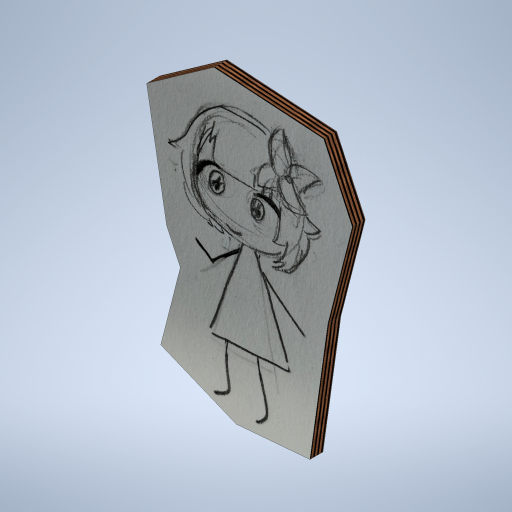
# Autodesk Inventor part: emu
Saved by Autodesk Inventor 2023 (Build 270158000, 158)
## iProperties
Created: 2024-07-02
Part Number: emu
Material: Generic
Document SubType Name: Modeling
Designer: Student-27
Density: 1 g/cm^3
Appearance: Default
Author: Student-27
Autodesk Inventor part; units mm, degrees
ref_plane "YZ Plane" through (0, 0, 0) normal (1, 0, 0) x (0, 1, 0)
ref_plane "XZ Plane" through (0, 0, 0) normal (0, 1, 0) x (-1, 0, 0)
ref_plane "XY Plane" through (0, 0, 0) normal (0, 0, 1) x (1, 0, 0)
sketch "Sketch1" plane through (0, 0, 0) normal (0, 0, 1) x (1, 0, 0)
  line L0 (-15.9123, 14.7509) -> (784.1877, 14.7509) construction
  line L1 (784.1877, 14.7509) -> (784.1877, -1052.0491) construction
  line L2 (784.1877, -1052.0491) -> (-15.9123, -1052.0491) construction
  line L3 (-15.9123, -1052.0491) -> (-15.9123, 14.7509) construction
  line L4 (311.9145, -258.6605) -> (525.4879, -272.6195)
  line L5 (525.4879, -272.6195) -> (581.2504, -393.4383)
  line L6 (581.2504, -393.4383) -> (533.62, -580.4751)
  line L7 (533.62, -580.4751) -> (498.7684, -826.7595)
  line L8 (498.7684, -826.7595) -> (355.243, -838.8475)
  line L9 (355.243, -838.8475) -> (208.3043, -778.5549)
  line L10 (208.3043, -778.5549) -> (246.337, -629.207)
  line L11 (246.337, -629.207) -> (219.57, -571.2118)
  line L12 (219.57, -571.2118) -> (180.7596, -351.4058)
  line L13 (180.7596, -351.4058) -> (311.9145, -258.6605)
  line L14 (180.7596, -258.6605) -> (584.1903, -258.6605)
  line L15 (584.1903, -258.6605) -> (584.1903, -838.8475)
  line L16 (584.1903, -838.8475) -> (180.7596, -838.8475)
  line L17 (180.7596, -838.8475) -> (180.7596, -258.6605)
  point P0 (0, 0)
  dimension "d7" = 403.4308
  dimension "d10" = 580.187
  constraints: 28 end point, 4 parallel, 1 horizontal, 1 perpendicular, 2 other
  measures "d7" distance of L14.start L14.end
  measures "d10" distance of L16.end L14.start
extrude "Extrusion1" add sketch "Sketch1" against normal blind 25.4 contours L4 L5 L6 L7 L8 L9 L10 L11 L12 L13
body "Solid1"
